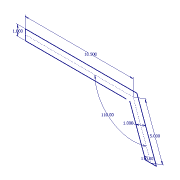
# Autodesk Inventor part: UpperArm
Saved by Autodesk Inventor 2012 (Build 160160000, 160)
## iProperties
Created: 2013-01-19
Part Number: UpperArm
Material: Aluminum-6061
Document SubType Name: Modeling
Designer: JesseK
Density: 2.71 g/cm^3
Author: JesseK
Autodesk Inventor part; units mm, degrees
ref_plane "YZ Plane" through (0, 0, 0) normal (1, 0, 0) x (0, 1, 0)
ref_plane "XZ Plane" through (0, 0, 0) normal (0, 1, 0) x (-1, 0, 0)
ref_plane "XY Plane" through (0, 0, 0) normal (0, 0, 1) x (1, 0, 0)
sketch "Sketch1" plane through (0, 0, 0) normal (0, 0, 1) x (1, 0, 0)
  line L0 (0, 0) -> (257.8074, 0)
  line L1 (275.5926, 25.4) -> (0, 25.4)
  line L2 (0, 25.4) -> (0, 0)
  line L3 (0, 12.7) -> (266.7, 12.7) construction
  line L4 (266.7, 12.7) -> (310.1366, -106.641) construction
  line L5 (275.5926, 25.4) -> (323.6516, -106.641)
  line L6 (323.6516, -106.641) -> (296.6215, -106.641)
  line L7 (296.6215, -106.641) -> (257.8074, 0)
  dimension "d4" = 25.4
  dimension "d5" = 110
  dimension "d6" = 266.7
  dimension "d7" = 127
  dimension "d17" = 110
  dimension "d18" = 25.4
  constraints: 16 end point, 3 parallel, 2 horizontal, 2 midpoint, 1 vertical
  measures "d4" distance of L1.end L0.start
  measures "d5" angle of L4 L3
  measures "d6" distance of L3.start L3.end
  measures "d7" distance of L3.end L4.end
  measures "d17" angle of L6 L7
  measures "d18" distance between parallel lines of L5 L7
extrude "Extrusion3" add sketch "Sketch1" along normal blind 25.4
shell "Shell3" thickness 1.5875 removed faces 2 at (0, 16.9333, 8.4667) at (305.6315, -106.641, 8.4667)
sketch "Sketch4" plane through (0, 0, 25.4) normal (0, 0, 1) x (1, 0, 0)
  line L0 (0, 0) -> (0, 25.4) projected
  line L1 (257.8074, 0) -> (0, 0) projected
  circle A0 centre (12.7, 12.7) radius 3.175
  dimension "d21" = 6.35
  dimension "d22" = 12.7
  dimension "d23" = 12.7
  constraints: 1 centre point
  measures "d21" diameter of A0
  measures "d22" distance from line of L1 A0.centre
  measures "d23" distance from line of L0 A0.centre
extrude "Extrusion4" cut sketch "Sketch4" against normal through all
fillet "Fillet2" radius 12.7 2 edges at (0, 0, 12.7) (0, 25.4, 12.7)
body "Solid2"
